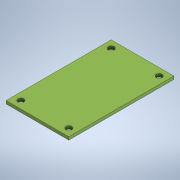
# Autodesk Inventor part: Status Indicator PCB
Saved by Autodesk Inventor 2021 (Build 250183000, 183)
## iProperties
Created: 2020-07-06
Part Number: Status Indicator PCB
Material: Generic
Document SubType Name: Modeling
Designer: jgray
Density: 1 g/cm^3
Appearance: Default
Author: jgray
Autodesk Inventor part; units mm, degrees
ref_plane "YZ Plane" through (0, 0, 0) normal (1, 0, 0) x (0, 1, 0)
ref_plane "XZ Plane" through (0, 0, 0) normal (0, 1, 0) x (-1, 0, 0)
ref_plane "XY Plane" through (0, 0, 0) normal (0, 0, 1) x (1, 0, 0)
sketch "Sketch1" plane through (0, 0, 0) normal (0, 1, 0) x (-1, 0, 0)
  line L0 (0, 0) -> (34, 0)
  line L1 (34, 0) -> (34, -57)
  line L2 (34, -57) -> (0, -57)
  line L3 (0, -57) -> (0, 0)
  line L4 (39.9452, -28.5) -> (-12.5583, -28.5) construction
  line L5 (17, 5.3263) -> (17, -64.2642) construction
  line L6 (4, -53) -> (30, -53) construction
  line L7 (30, -53) -> (30, -4) construction
  line L8 (30, -4) -> (4, -4) construction
  line L9 (4, -4) -> (4, -53) construction
  line L10 (4, -53) -> (30, -4) construction
  line L11 (30, -53) -> (4, -4) construction
  circle A0 centre (30, -4) radius 1.6
  circle A1 centre (30, -53) radius 1.6
  circle A2 centre (4, -4) radius 1.6
  circle A3 centre (4, -53) radius 1.6
  point P0 (34, -28.5)
  point P1 (17, -57)
  point P2 (17, -28.5)
  dimension "d0" = 34
  dimension "d1" = 57
  dimension "d2" = 26
  dimension "d3" = 49
  dimension "d4" = 3.2
  dimension "d5" = 3.2
  dimension "d6" = 3.2
  dimension "d7" = 3.2
  constraints: 24 end point, 4 centre point, 4 coincident, 4 midpoint, 4 parallel, 4 point on line, 3 horizontal, 2 perpendicular, 1 vertical
  measures "d0" distance of L1.end L2.end
  measures "d1" distance of L0.end L1.end
  measures "d2" distance of L8.end L7.end
  measures "d3" distance of L7.end L6.end
  measures "d4" diameter of A0
  measures "d5" diameter of A1
  measures "d6" diameter of A2
  measures "d7" diameter of A3
extrude "Extrusion1" add sketch "Sketch1" along normal blind 1.65
body "Solid1"
